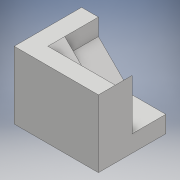
# Autodesk Inventor part: 19
Saved by Autodesk Inventor 2017 (Build 210142000, 142)
## iProperties
Part Number: 19
Material: 一般
Document SubType Name: Modeling
Designer: Brian
Density: 1 g/cm^3
Appearance: 預設
Author: Brian
Autodesk Inventor part; units mm, degrees
ref_plane "YZ Plane" through (0, 0, 0) normal (1, 0, 0) x (0, 1, 0)
ref_plane "XZ Plane" through (0, 0, 0) normal (0, 1, 0) x (-1, 0, 0)
ref_plane "XY Plane" through (0, 0, 0) normal (0, 0, 1) x (1, 0, 0)
sketch "草圖1" plane through (0, 0, 0) normal (0, 1, 0) x (-1, 0, 0)
  line L0 (0, 0) -> (-50, 0)
  line L1 (-50, 0) -> (-50, -40)
  line L2 (-50, -40) -> (0, -40)
  line L3 (0, -40) -> (0, 0)
  dimension "d0" = 50
  dimension "d1" = 40
  constraints: 8 end point, 2 parallel, 1 horizontal, 1 perpendicular
  measures "d0" distance of L1.end L2.end
  measures "d1" distance of L2.end L0.start
extrude "擠出1" add sketch "草圖1" along normal blind 40
sketch "草圖2" plane through (0, 40, 0) normal (0, 1, 0) x (1, 0, 0)
  line L0 (0, 0) -> (50, 0) projected
  line L1 (50, 0) -> (10, 0)
  line L2 (10, 0) -> (10, 30)
  line L3 (10, 30) -> (50, 30)
  line L4 (50, 30) -> (50, 0)
  dimension "d4" = 40
  dimension "d5" = 30
  constraints: 8 end point, 2 parallel, 1 horizontal, 1 perpendicular
  measures "d4" distance of L2.end L3.end
  measures "d5" distance of L1.end L2.end
extrude "擠出2" cut sketch "草圖2" against normal blind 10
chamfer "倒角1" distance 10 angle 45 1 edges at (10, 35, -30)
sketch "草圖3" plane through (0, 30, 0) normal (0, 1, 0) x (1, 0, 0)
  line L0 (50, 30) -> (50, 0) projected
  line L1 (50, 0) -> (10, 0)
  line L2 (10, 0) -> (10, 30)
  line L3 (10, 30) -> (50, 30)
  line L4 (50, 30) -> (50, 0)
  point P0 (0, 0)
  constraints: 8 end point, 2 parallel, 1 horizontal, 1 perpendicular
extrude "擠出3" cut sketch "草圖3" against normal blind 10
chamfer "倒角2" distance 20 angle 45 1 edges at (10, 25, -30)
sketch "草圖4" plane through (0, 20, 0) normal (0, 1, 0) x (1, 0, 0)
  line L0 (50, 0) -> (10, 0) projected
  line L1 (50, 0) -> (30, 20)
  line L2 (0, 0) -> (10, 0) projected
  line L3 (30, 20) -> (10, 0)
  dimension "d16" = 45
  constraints: 4 end point, 1 perpendicular
  measures "d16" angle of L0 L3
extrude "擠出4" cut sketch "草圖4" against normal blind 10
